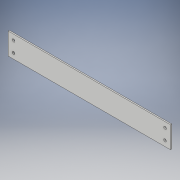
# Autodesk Inventor part: slider-crossbeam
Saved by Autodesk Inventor 2017 (Build 210142000, 142)
## iProperties
Created: 2017-12-27
Part Number: slider-crossbeam
Material: Generic
Document SubType Name: Modeling
Designer: Micah
Density: 1 g/cm^3
Appearance: Default
Author: Micah
Autodesk Inventor part; units mm, degrees
ref_plane "YZ Plane" through (0, 0, 0) normal (1, 0, 0) x (0, 1, 0)
ref_plane "XZ Plane" through (0, 0, 0) normal (0, 1, 0) x (-1, 0, 0)
ref_plane "XY Plane" through (0, 0, 0) normal (0, 0, 1) x (1, 0, 0)
sketch "Sketch1" plane through (0, 0, 0) normal (0, 0, 1) x (1, 0, 0)
  line L0 (0, 0) -> (381, 0)
  line L1 (381, 0) -> (381, 50.8)
  line L2 (381, 50.8) -> (0, 50.8)
  line L3 (0, 50.8) -> (0, 0)
  line L4 (12.7, 50.8) -> (12.7, 0) construction
  line L5 (0, 38.1) -> (12.7, 38.1) construction
  line L6 (0, 12.7) -> (12.7, 12.7) construction
  circle A0 centre (12.7, 38.1) radius 3.175
  circle A1 centre (12.7, 12.7) radius 3.175
  line L7 (190.5, 50.8) -> (190.5, 0) construction
  line L8 (368.3, 50.8) -> (368.3, 0) construction
  line L9 (381, 38.1) -> (368.3, 38.1) construction
  line L10 (381, 12.7) -> (368.3, 12.7) construction
  circle A2 centre (368.3, 38.1) radius 3.175
  circle A3 centre (368.3, 12.7) radius 3.175
  dimension "d0" = 381
  dimension "d1" = 50.8
  dimension "d2" = 12.7
  dimension "d3" = 12.7
  dimension "d4" = 25.4
  dimension "d5" = 6.35
  dimension "d6" = 6.35
  constraints: 22 end point, 8 point on line, 8 symmetric about line, 4 centre point, 4 coincident, 4 perpendicular, 2 midpoint, 2 parallel, 1 horizontal, 2 other
  measures "d0" distance of L2.end L1.end
  measures "d1" distance of L1.end L0.end
  measures "d2" distance between parallel lines of L4 L3
  measures "d3" distance between parallel lines of L2 L5
  measures "d4" distance between parallel lines of L6 L5
  measures "d5" diameter of A0
  measures "d6" diameter of A1
extrude "Extrusion1" add sketch "Sketch1" along normal blind 3.175
body "Solid1"
